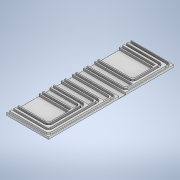
# Autodesk Inventor part: wire_holder_half2
Saved by Autodesk Inventor 2021 (Build 250183000, 183)
## iProperties
Created: 2021-02-03
Part Number: wire_holder_half2
Material: Generic
Document SubType Name: Modeling
Designer: User
Density: 1 g/cm^3
Appearance: Default
Author: User
Autodesk Inventor part; units mm, degrees
ref_plane "YZ Plane" through (0, 0, 0) normal (1, 0, 0) x (0, 1, 0)
ref_plane "XZ Plane" through (0, 0, 0) normal (0, 1, 0) x (-1, 0, 0)
ref_plane "XY Plane" through (0, 0, 0) normal (0, 0, 1) x (1, 0, 0)
sketch "Sketch1" plane through (0, 0, 0) normal (0, 1, 0) x (-1, 0, 0)
  line L0 (-418.4221, -16) -> (-508.4221, -16)
  line L1 (-518.4221, -6) -> (-518.4221, 140)
  line L2 (-508.4221, 150) -> (-418.4221, 150)
  line L3 (-418.4221, -11) -> (-508.4221, -11)
  line L4 (-513.4221, -6) -> (-513.4221, 140)
  line L5 (-508.4221, 145) -> (-418.4221, 145)
  line L6 (-418.4221, 16) -> (-498.4221, 16)
  line L7 (-503.4221, 21) -> (-503.4221, 130)
  line L8 (-418.4221, 11) -> (-498.4221, 11)
  line L9 (-508.4221, 21) -> (-508.4221, 130)
  line L10 (-498.4221, 135) -> (-418.4221, 135)
  line L11 (-498.4221, 140) -> (-418.4221, 140)
  line L12 (-418.4221, 43) -> (-488.4221, 43)
  line L13 (-418.4221, 38) -> (-488.4221, 38)
  line L14 (-493.4221, 48) -> (-493.4221, 120)
  line L15 (-488.4221, 125) -> (-418.4221, 125)
  line L16 (-418.4221, 70) -> (-488.4221, 70)
  line L17 (-498.4221, 48) -> (-498.4221, 120)
  line L18 (-488.4221, 130) -> (-418.4221, 130)
  line L19 (-418.4221, 65) -> (-488.4221, 65)
  line L20 (-488.4221, 70) -> (-488.4221, 65)
  line L21 (-418.4221, -150) -> (-508.4221, -150)
  line L22 (-518.4221, -140) -> (-518.4221, -48)
  line L23 (-418.4221, -145) -> (-508.4221, -145)
  line L24 (-508.4221, -38) -> (-418.4221, -38)
  line L25 (-418.4221, -140) -> (-498.4221, -140)
  line L26 (-513.4221, -140) -> (-513.4221, -48)
  line L27 (-508.4221, -43) -> (-418.4221, -43)
  line L28 (-418.4221, -135) -> (-498.4221, -135)
  line L29 (-503.4221, -130) -> (-503.4221, -75)
  line L30 (-508.4221, -130) -> (-508.4221, -75)
  line L31 (-498.4221, -65) -> (-418.4221, -65)
  line L32 (-498.4221, -70) -> (-418.4221, -70)
  line L33 (-418.4221, -125) -> (-498.4221, -125)
  line L34 (-418.4221, -130) -> (-498.4221, -130)
  line L35 (-498.4221, -130) -> (-498.4221, -125)
  line L36 (-528.4221, -160) -> (-528.4221, 160)
  line L37 (-418.4221, -160) -> (-528.4221, -160)
  line L38 (-528.4221, 160) -> (-418.4221, 160)
  line L39 (-418.4221, -221.6121) -> (-418.4221, 308.2529) construction
  line L40 (-418.4221, -160) -> (-418.4221, 160)
  line L41 (-418.4221, -122) -> (-500.4221, -122)
  line L42 (-500.4221, -122) -> (-500.4221, -78)
  line L43 (-495.4221, -73) -> (-418.4221, -73)
  line L44 (-418.4221, -73) -> (-418.4221, -122)
  line L45 (-505.4221, -62) -> (-418.4221, -62)
  line L46 (-418.4221, -62) -> (-418.4221, -46)
  line L47 (-418.4221, -46) -> (-505.4221, -46)
  line L48 (-510.4221, -51) -> (-510.4221, -57)
  line L49 (-522.4221, -35) -> (-418.4221, -35)
  line L50 (-418.4221, -35) -> (-418.4221, -19)
  line L51 (-418.4221, -19) -> (-522.4221, -19)
  line L52 (-522.4221, -19) -> (-522.4221, -35)
  line L53 (-505.4221, -8) -> (-418.4221, -8)
  line L54 (-418.4221, -8) -> (-418.4221, 8)
  line L55 (-418.4221, 8) -> (-510.4221, 8)
  line L56 (-510.4221, 8) -> (-510.4221, -3)
  line L57 (-495.4221, 19) -> (-418.4221, 19)
  line L58 (-418.4221, 19) -> (-418.4221, 35)
  line L59 (-418.4221, 35) -> (-500.4221, 35)
  line L60 (-500.4221, 35) -> (-500.4221, 24)
  line L61 (-490.4221, 73) -> (-418.4221, 73)
  line L62 (-418.4221, 73) -> (-418.4221, 122)
  line L63 (-418.4221, 122) -> (-485.4221, 122)
  line L64 (-490.4221, 117) -> (-490.4221, 73)
  line L65 (-485.4221, 47.0076) -> (-418.4221, 47.0076)
  line L66 (-418.4221, 47.0076) -> (-418.4221, 61.4689)
  line L67 (-418.4221, 61.4689) -> (-490.4221, 61.4689)
  line L68 (-490.4221, 61.4689) -> (-490.4221, 52.0076)
  arc A0 (-503.4221, -130) -> (-498.4221, -135) centre (-498.4221, -130) ccw
  arc A1 (-498.4221, -70) -> (-503.4221, -75) centre (-498.4221, -75) ccw
  arc A2 (-513.4221, -140) -> (-508.4221, -145) centre (-508.4221, -140) ccw
  arc A3 (-505.4221, -46) -> (-510.4221, -51) centre (-505.4221, -51) ccw
  arc A4 (-508.4221, -43) -> (-513.4221, -48) centre (-508.4221, -48) ccw
  arc A5 (-508.4221, -130) -> (-498.4221, -140) centre (-498.4221, -130) ccw
  arc A6 (-498.4221, -65) -> (-508.4221, -75) centre (-498.4221, -75) ccw
  arc A7 (-493.4221, 48) -> (-488.4221, 43) centre (-488.4221, 48) ccw
  arc A8 (-488.4221, 125) -> (-493.4221, 120) centre (-488.4221, 120) ccw
  arc A9 (-485.4221, 122) -> (-490.4221, 117) centre (-485.4221, 117) ccw
  arc A10 (-490.4221, 52.0076) -> (-485.4221, 47.0076) centre (-485.4221, 52.0076) ccw
  arc A11 (-498.4221, 48) -> (-488.4221, 38) centre (-488.4221, 48) ccw
  arc A12 (-488.4221, 130) -> (-498.4221, 120) centre (-488.4221, 120) ccw
  arc A13 (-498.4221, 140) -> (-508.4221, 130) centre (-498.4221, 130) ccw
  arc A14 (-508.4221, 21) -> (-498.4221, 11) centre (-498.4221, 21) ccw
  arc A15 (-503.4221, 21) -> (-498.4221, 16) centre (-498.4221, 21) ccw
  arc A16 (-498.4221, 135) -> (-503.4221, 130) centre (-498.4221, 130) ccw
  arc A17 (-508.4221, 145) -> (-513.4221, 140) centre (-508.4221, 140) ccw
  arc A18 (-510.4221, -3) -> (-505.4221, -8) centre (-505.4221, -3) ccw
  arc A19 (-513.4221, -6) -> (-508.4221, -11) centre (-508.4221, -6) ccw
  arc A20 (-518.4221, -6) -> (-508.4221, -16) centre (-508.4221, -6) ccw
  arc A21 (-508.4221, 150) -> (-518.4221, 140) centre (-508.4221, 140) ccw
  arc A22 (-495.4221, -73) -> (-500.4221, -78) centre (-495.4221, -78) ccw
  arc A23 (-500.4221, 24) -> (-495.4221, 19) centre (-495.4221, 24) ccw
  line L69 (-508.4221, -160) -> (-508.4221, -140) construction
  line L70 (-508.4221, -140) -> (-528.4221, -140) construction
  arc A24 (-518.4221, -140) -> (-508.4221, -150) centre (-508.4221, -140) ccw
  line L71 (-508.4221, -38) -> (-508.4221, -43) construction
  arc A25 (-508.4221, -38) -> (-518.4221, -48) centre (-508.4221, -48) ccw
  line L72 (-510.4221, -57) -> (-510.4221, -62)
  line L73 (-505.4221, -62) -> (-510.4221, -62)
  point P0 (-518.4221, -16)
  point P1 (-518.4221, 150)
  point P2 (-513.4221, -11)
  point P3 (-513.4221, 145)
  point P4 (-503.4221, 16)
  point P5 (-503.4221, 135)
  point P6 (-508.4221, 11)
  point P7 (-493.4221, 43)
  point P8 (-498.4221, 38)
  point P9 (-493.4221, 125)
  point P10 (-498.4221, 130)
  point P11 (-508.4221, -150)
  point P12 (-513.4221, -145)
  point P13 (-508.4221, -140)
  point P14 (-513.4221, -43)
  point P15 (-503.4221, -135)
  point P16 (-503.4221, -70)
  point P17 (-508.4221, -65)
  point P18 (-518.4221, -94)
  point P19 (-500.4221, -73)
  point P20 (-510.4221, -46)
  point P21 (-510.4221, -8)
  point P22 (-500.4221, 19)
  point P23 (-490.4221, 122)
  point P24 (-490.4221, 47.0076)
  point P25 (-518.4221, -140)
  point P26 (-518.4221, -43)
  dimension "d2" = 5
  dimension "d3" = 5
  dimension "d5" = 5
  dimension "d6" = 5
  dimension "d7" = 5
  dimension "d9" = 5
  dimension "d12" = 22
  dimension "d13" = 5
  dimension "d14" = 5
  dimension "d15" = 22
  dimension "d16" = 5
  dimension "d17" = 5
  dimension "d18" = 5
  dimension "d20" = 22
  dimension "d22" = 5
  dimension "d23" = 5
  dimension "d24" = 5
  dimension "d32" = 5
  dimension "d35" = 5
  dimension "d38" = 5
  dimension "d40" = 5
  dimension "d41" = 5
  dimension "d42" = 5
  dimension "d43" = 5
  dimension "d46" = 22
  dimension "d47" = 5
  dimension "d48" = 5
  dimension "d49" = 5
  dimension "d50" = 5
  dimension "d61" = 10
  dimension "d62" = 10
  dimension "d63" = 110
  dimension "d64" = 3
  dimension "d65" = 3
  dimension "d66" = 3
  dimension "d67" = 3
  dimension "d68" = 3
  dimension "d69" = 3
  dimension "d70" = 3
  dimension "d71" = 3
  dimension "d72" = 6
  dimension "d73" = 3
  dimension "d74" = 3
  dimension "d75" = 3
  dimension "d76" = 3
  dimension "d77" = 3
  dimension "d78" = 3
  dimension "d79" = 3
  dimension "d80" = 3
  dimension "d81" = 3
  dimension "d87" = 5
  dimension "d88" = 10
  dimension "d89" = 5
  dimension "d90" = 10
  dimension "d91" = 5
  dimension "d92" = 10
  dimension "d93" = 10
  constraints: 144 end point, 58 point on line, 52 point on circle, 52 tangent, 26 centre point, 22 perpendicular, 20 horizontal, 20 parallel, 17 equal radius, 6 vertical, 3 midpoint, 40 other
  measures "d2" distance between parallel lines of L1 L4
  measures "d3" distance between parallel lines of L2 L5
  measures "d5" distance between parallel lines of L11 L5
  measures "d6" distance between parallel lines of L4 L9
  measures "d7" distance between parallel lines of L8 L6
  measures "d9" distance between parallel lines of L11 L10
  measures "d12" distance between parallel lines of L3 L8
  measures "d13" distance between parallel lines of L9 L7
  measures "d14" distance between parallel lines of L13 L12
  measures "d15" distance between parallel lines of L6 L13
  measures "d16" distance between parallel lines of L10 L18
  measures "d17" distance between parallel lines of L7 L17
  measures "d18" distance between parallel lines of L18 L15
  measures "d20" distance between parallel lines of L12 L19
  measures "d22" distance between parallel lines of L19 L16
  measures "d23" distance between parallel lines of L17 L14
  measures "d24" distance between parallel lines of L14 L20
  measures "d32" distance between parallel lines of L21 L23
  measures "d35" distance between parallel lines of L22 L26
  measures "d38" distance between parallel lines of L24 L27
  measures "d40" distance between parallel lines of L25 L28
  measures "d41" distance between parallel lines of L23 L25
  measures "d42" distance between parallel lines of L30 L29
  measures "d43" distance between parallel lines of L31 L32
  measures "d46" distance between parallel lines of L31 L27
  measures "d47" distance between parallel lines of L26 L30
  measures "d48" distance between parallel lines of L34 L33
  measures "d49" distance between parallel lines of L28 L34
  measures "d50" distance between parallel lines of L29 L35
  measures "d61" distance between parallel lines of L36 L22
  measures "d62" distance between parallel lines of L36 L1
  measures "d64" distance between parallel lines of L29 L42
  measures "d65" distance between parallel lines of L43 L32
  measures "d66" distance between parallel lines of L41 L33
  measures "d67" distance between parallel lines of L31 L45
  measures "d68" distance between parallel lines of L27 L47
  measures "d69" distance between parallel lines of L26 L48
  measures "d70" distance between parallel lines of L24 L49
  measures "d71" distance between parallel lines of L0 L51
  measures "d72" distance between parallel lines of L52 L36
  measures "d73" distance between parallel lines of L3 L53
  measures "d74" distance between parallel lines of L8 L55
  measures "d75" distance between parallel lines of L4 L56
  measures "d76" distance between parallel lines of L7 L60
  measures "d77" distance between parallel lines of L6 L57
  measures "d78" distance between parallel lines of L13 L59
  measures "d79" distance between parallel lines of L14 L68
  measures "d80" distance between parallel lines of L16 L61
  measures "d81" distance between parallel lines of L15 L63
  measures "d87" radius of A0
  measures "d88" radius of A5
  measures "d89" radius of A7
  measures "d90" radius of A11
  measures "d91" radius of A23
  measures "d92" radius of A24
  measures "d93" radius of A25
extrude "Extrusion1" add sketch "Sketch1" along normal blind 5 contours L40 L51 L52 L49 L24 A25 L22 A24 L21 L37 L36 L38 L2 A21 L1 A20 L0 | L3 A19 L4 A17 L5 L40 L11 A13 L9 A14 L8 L55 L56 A18 L53 | L40 L47 A3 L48 L72 L73 L45 L31 A6 L30 A5 L25 L23 A2 L26 A4 L27 | L6 A15 L7 A16 L10 L40 L18 A12 L17 A11 L13 L59 L60 A23 L57 | L40 L43 A22 L42 L41 L33 L35 L34 L28 A0 L29 A1 L32 | L12 A7 L14 A8 L15 L40 L63 A9 L64 L61 L16 L20 L19 L67 L68 A10 L65
sketch "Sketch2" plane through (528.4221, 0, -160) normal (0, 0, -1) x (-1, 0, 0)
  line L0 (0, 0) -> (0, 5) projected
  line L1 (0, 0) -> (110, 0)
  line L2 (110, 0) -> (110, -0.5)
  line L3 (110, -0.5) -> (0, -0.5)
  line L4 (0, -0.5) -> (0, 0)
  point P0 (528.4221, 0)
  dimension "d84" = 0.5
  constraints: 8 end point, 2 parallel, 1 horizontal, 1 perpendicular
  measures "d84" distance of L3.end L0.start
extrude "Extrusion2" add sketch "Sketch2" against normal blind 320
sketch "Sketch3" plane through (418.4221, 0, -130) normal (0, 1, 0) x (1, 0, 0)
  line L0 (0, 0) -> (80, 0) projected
  line L1 (80, -5) -> (0, -5) projected
  line L2 (80, 0) -> (70, 0)
  line L3 (70, 0) -> (70, -5)
  line L4 (70, -5) -> (80, -5)
  line L5 (80, -5) -> (80, 0)
  line L6 (70, -200) -> (0, -200) projected
  line L7 (70, -194.9709) -> (60, -194.9709)
  line L8 (60, -194.9709) -> (60, -200)
  line L9 (60, -200) -> (70, -200)
  line L10 (70, -200) -> (70, -194.9709)
  point P0 (-418.4221, -130)
  dimension "d94" = 10
  dimension "d95" = 10
  constraints: 16 end point, 4 parallel, 3 point on line, 2 horizontal, 2 perpendicular
  measures "d94" distance of L4.end L3.end
  measures "d95" distance of L9.end L8.end
extrude "Extrusion3" cut sketch "Sketch3" against normal blind 15
sketch "Sketch4" plane through (0, 5, 0) normal (0, 1, 0) x (1, 0, 0)
  line L0 (418.4221, 160) -> (418.4221, -160) projected
  line L1 (418.4221, 152) -> (520.4221, 152)
  line L2 (520.4221, 152) -> (520.4221, -152)
  line L3 (520.4221, -152) -> (418.4221, -152)
  line L4 (418.4221, -152) -> (418.4221, 152)
  line L5 (518.4221, 6) -> (518.4221, -140) projected
  line L6 (508.4221, -150) -> (418.4221, -150) projected
  line L7 (418.4221, 150) -> (508.4221, 150) projected
  line L8 (528.4221, 160) -> (528.4221, -160) projected
  line L9 (528.4221, 160) -> (418.4221, 160)
  line L10 (418.4221, 160) -> (418.4221, -160)
  line L11 (418.4221, -160) -> (528.4221, -160)
  line L12 (528.4221, -160) -> (528.4221, 160)
  point P0 (0, 0)
  dimension "d98" = 2
  dimension "d99" = 2
  dimension "d100" = 2
  constraints: 16 end point, 4 parallel, 2 horizontal, 2 perpendicular, 1 point on line
  measures "d98" distance between parallel lines of L2 L5
  measures "d99" distance between parallel lines of L6 L3
  measures "d100" distance between parallel lines of L1 L7
extrude "Extrusion4" cut sketch "Sketch4" against normal blind 10 contours L9 L8 L11 L0 L3 L2 L1
equation "\"d2\" = d25"
equation "\"d3\" = d25"
equation "\"d5\" = d26"
equation "\"d6\" = d26"
equation "\"d7\" = d25"
equation "\"d9\" = d25"
equation "\"d12\" = d28"
equation "\"d13\" = d25"
equation "\"d14\" = d25"
equation "\"d15\" = d28"
equation "\"d16\" = d26"
equation "\"d17\" = d26"
equation "\"d18\" = d25"
equation "\"d20\" = d28"
equation "\"d22\" = d25"
equation "\"d23\" = d25"
equation "\"d24\" = d26"
equation "\"d32\" = d51"
equation "\"d35\" = d51"
equation "\"d38\" = d51"
equation "\"d40\" = d51"
equation "\"d41\" = d53"
equation "\"d42\" = d51"
equation "\"d43\" = d51"
equation "\"d46\" = d54"
equation "\"d47\" = d53"
equation "\"d48\" = d51"
equation "\"d49\" = d53"
equation "\"d50\" = d53"
equation "\"d25\" = 5"
equation "\"d26\" = 5"
equation "\"d28\" = -1.2 * d25 + 0.2 * d29"
equation "\"d51\" = 5"
equation "\"d53\" = 5"
equation "\"d54\" = -1.2 * d51 + 0.2 * d55"
equation "\"d29\" = 140"
equation "\"d55\" = 140"
body "Solid1"
